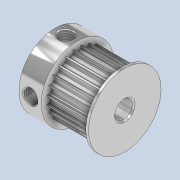
# Autodesk Inventor part: M6.35 24Tooth 15mm Deep 3M Timing Pulley
Saved by Autodesk Inventor 2022 (Build 260153000, 153)
## iProperties
Created: 2021-10-10
Part Number: M6.35 24Tooth 15mm Deep 3M Timing Pulley
Material: Generic
Document SubType Name: Modeling
Designer: Coy
Density: 1 g/cm^3
Appearance: Chrome - Polished
Author: Coy
Autodesk Inventor part; units mm, degrees
ref_plane "YZ Plane" through (0, 0, 0) normal (1, 0, 0) x (0, 1, 0)
sketch "Sketch1" plane through (0, 0, 0) normal (1, 0, 0) x (0, 1, 0)
  circle A0 centre (0, 0) radius 3.175
  circle A1 centre (0, 0) radius 13
  dimension "d0" = 6.35
  dimension "d1" = 26
  constraints: 2 centre point, 2 coincident
  measures "d0" diameter of A0
  measures "d1" diameter of A1
extrude "Extrusion1" add sketch "Sketch1" along normal blind 8
sketch "Sketch2" plane through (8, 0, 0) normal (1, 0, 0) x (0, 0, -1)
  circle A0 centre (0, 0) radius 3.175
  circle A1 centre (0, 0) radius 11.08
  line L0 (-1.45, 14.5114) -> (-1.45, 7.0707) construction
  line L1 (1.45, 14.5114) -> (1.45, 7.0707) construction
  arc A2 (-1.2, 10.18) -> (1.2, 10.18) centre (0, 11.08) ccw
  line L2 (1.2, 11.0148) -> (1.2, 10.18)
  line L3 (-1.2, 11.0148) -> (-1.2, 10.18)
  line L4 (-4.01, 10.3289) -> (-3.7939, 9.5225)
  arc A3 (-3.7939, 9.5225) -> (-1.4757, 10.1437) centre (-2.8677, 10.7025) ccw
  line L5 (-1.6917, 10.9501) -> (-1.4757, 10.1437)
  line L6 (-6.5466, 8.9391) -> (-6.1292, 8.2161)
  arc A4 (-6.1292, 8.2161) -> (-4.0508, 9.4161) centre (-5.54, 9.5956) ccw
  line L7 (-4.4682, 10.1391) -> (-4.0508, 9.4161)
  line L8 (-8.6372, 6.9401) -> (-8.0469, 6.3498)
  arc A5 (-8.0469, 6.3498) -> (-6.3498, 8.0469) centre (-7.8347, 7.8347) ccw
  line L9 (-6.9401, 8.6372) -> (-6.3498, 8.0469)
  line L10 (-10.1391, 4.4682) -> (-9.4161, 4.0508)
  arc A6 (-9.4161, 4.0508) -> (-8.2161, 6.1292) centre (-9.5956, 5.54) ccw
  line L11 (-8.9391, 6.5466) -> (-8.2161, 6.1292)
  line L12 (-10.9501, 1.6917) -> (-10.1437, 1.4757)
  arc A7 (-10.1437, 1.4757) -> (-9.5225, 3.7939) centre (-10.7025, 2.8677) ccw
  line L13 (-10.3289, 4.01) -> (-9.5225, 3.7939)
  line L14 (-11.0148, -1.2) -> (-10.18, -1.2)
  arc A8 (-10.18, -1.2) -> (-10.18, 1.2) centre (-11.08, 0) ccw
  line L15 (-11.0148, 1.2) -> (-10.18, 1.2)
  line L16 (-10.3289, -4.01) -> (-9.5225, -3.7939)
  arc A9 (-9.5225, -3.7939) -> (-10.1437, -1.4757) centre (-10.7025, -2.8677) ccw
  line L17 (-10.9501, -1.6917) -> (-10.1437, -1.4757)
  line L18 (-8.9391, -6.5466) -> (-8.2161, -6.1292)
  arc A10 (-8.2161, -6.1292) -> (-9.4161, -4.0508) centre (-9.5956, -5.54) ccw
  line L19 (-10.1391, -4.4682) -> (-9.4161, -4.0508)
  line L20 (-6.9401, -8.6372) -> (-6.3498, -8.0469)
  arc A11 (-6.3498, -8.0469) -> (-8.0469, -6.3498) centre (-7.8347, -7.8347) ccw
  line L21 (-8.6372, -6.9401) -> (-8.0469, -6.3498)
  line L22 (-4.4682, -10.1391) -> (-4.0508, -9.4161)
  arc A12 (-4.0508, -9.4161) -> (-6.1292, -8.2161) centre (-5.54, -9.5956) ccw
  line L23 (-6.5466, -8.9391) -> (-6.1292, -8.2161)
  line L24 (-1.6917, -10.9501) -> (-1.4757, -10.1437)
  arc A13 (-1.4757, -10.1437) -> (-3.7939, -9.5225) centre (-2.8677, -10.7025) ccw
  line L25 (-4.01, -10.3289) -> (-3.7939, -9.5225)
  line L26 (1.2, -11.0148) -> (1.2, -10.18)
  arc A14 (1.2, -10.18) -> (-1.2, -10.18) centre (0, -11.08) ccw
  line L27 (-1.2, -11.0148) -> (-1.2, -10.18)
  line L28 (4.01, -10.3289) -> (3.7939, -9.5225)
  arc A15 (3.7939, -9.5225) -> (1.4757, -10.1437) centre (2.8677, -10.7025) ccw
  line L29 (1.6917, -10.9501) -> (1.4757, -10.1437)
  line L30 (6.5466, -8.9391) -> (6.1292, -8.2161)
  arc A16 (6.1292, -8.2161) -> (4.0508, -9.4161) centre (5.54, -9.5956) ccw
  line L31 (4.4682, -10.1391) -> (4.0508, -9.4161)
  line L32 (8.6372, -6.9401) -> (8.0469, -6.3498)
  arc A17 (8.0469, -6.3498) -> (6.3498, -8.0469) centre (7.8347, -7.8347) ccw
  line L33 (6.9401, -8.6372) -> (6.3498, -8.0469)
  line L34 (10.1391, -4.4682) -> (9.4161, -4.0508)
  arc A18 (9.4161, -4.0508) -> (8.2161, -6.1292) centre (9.5956, -5.54) ccw
  line L35 (8.9391, -6.5466) -> (8.2161, -6.1292)
  line L36 (10.9501, -1.6917) -> (10.1437, -1.4757)
  arc A19 (10.1437, -1.4757) -> (9.5225, -3.7939) centre (10.7025, -2.8677) ccw
  line L37 (10.3289, -4.01) -> (9.5225, -3.7939)
  line L38 (11.0148, 1.2) -> (10.18, 1.2)
  arc A20 (10.18, 1.2) -> (10.18, -1.2) centre (11.08, 0) ccw
  line L39 (11.0148, -1.2) -> (10.18, -1.2)
  line L40 (10.3289, 4.01) -> (9.5225, 3.7939)
  arc A21 (9.5225, 3.7939) -> (10.1437, 1.4757) centre (10.7025, 2.8677) ccw
  line L41 (10.9501, 1.6917) -> (10.1437, 1.4757)
  line L42 (8.9391, 6.5466) -> (8.2161, 6.1292)
  arc A22 (8.2161, 6.1292) -> (9.4161, 4.0508) centre (9.5956, 5.54) ccw
  line L43 (10.1391, 4.4682) -> (9.4161, 4.0508)
  line L44 (6.9401, 8.6372) -> (6.3498, 8.0469)
  arc A23 (6.3498, 8.0469) -> (8.0469, 6.3498) centre (7.8347, 7.8347) ccw
  line L45 (8.6372, 6.9401) -> (8.0469, 6.3498)
  line L46 (4.4682, 10.1391) -> (4.0508, 9.4161)
  arc A24 (4.0508, 9.4161) -> (6.1292, 8.2161) centre (5.54, 9.5956) ccw
  line L47 (6.5466, 8.9391) -> (6.1292, 8.2161)
  line L48 (1.6917, 10.9501) -> (1.4757, 10.1437)
  arc A25 (1.4757, 10.1437) -> (3.7939, 9.5225) centre (2.8677, 10.7025) ccw
  line L49 (4.01, 10.3289) -> (3.7939, 9.5225)
  dimension "d4" = 22.16
  dimension "d5" = 1.45
  dimension "d6" = 1.45
  dimension "d7" = 3
  dimension "d8" = 0.25
  dimension "d9" = 0.25
  dimension "d10" = 11.08
  dimension "d13" = 360
  constraints: 100 end point, 48 point on circle, 25 centre point, 2 coincident, 2 parallel, 2 vertical, 197 other
  measures "d5" distance from line of point (0, 0) L1
  measures "d6" distance from line of point (0, 0) L0
  measures "d7" diameter of A2
  measures "d8" distance between parallel lines of L1 L2
  measures "d9" distance between parallel lines of L0 L3
  measures "d10" distance of point (0, 0) A2.centre
extrude "Extrusion2" add sketch "Sketch2" along normal blind 16 contours L38 A20 L39 A1 L36 A19 L37 L34 A18 L35 L32 A17 L33 L30 A16 L31 L28 A15 L29 L26 A14 L27 L24 A13 L25 L22 A12 L23 L20 A11 L21 L18 A10 L19 L16 A9 L17 L14 A8 L15 L12 A7 L13 L10 A6 L11 L8 A5 L9 L6 A4 L7 L4 A3 L5 L3 A2 L2 L48 A25 L49 L46 A24 L47 L44 A23 L45 L42 A22 L43 L40 A21 L41
sketch "Sketch3" plane through (24, 0, 0) normal (1, 0, 0) x (0, 0, -1)
  circle A0 centre (0, 0) radius 13 projected
  circle A1 centre (0, 0) radius 3.175 projected
extrude "Extrusion3" add sketch "Sketch3" along normal blind 1
chamfer "Chamfer1" distance 0.5 angle 45 2 edges at (25, 0, 3.175) (0, -3.175, 0)
ref_plane "Work Plane1" through (0, 13, 0) normal (0, 1, 0) x (-1, 0, 0)
sketch "Sketch4" plane through (0, 13, 0) normal (0, 1, 0) x (-1, 0, 0)
  line L0 (0, 0) -> (-8, 0) construction
  line L1 (-8, 13) -> (-8, -13) construction
  circle A0 centre (-4, 0) radius 2.5
  dimension "d23" = 5
  constraints: 2 end point, 2 midpoint, 1 centre point
  measures "d23" diameter of A0
extrude "Extrusion4" cut sketch "Sketch4" against normal up to next
ref_plane "Work Plane2" through (0, 0, 13) normal (0, 0, 1) x (1, 0, 0)
sketch "Sketch5" plane through (0, 0, 13) normal (0, 0, 1) x (1, 0, 0)
  line L0 (0, 0) -> (8, 0) construction
  line L1 (8, -13) -> (8, 13) construction
  circle A0 centre (4, 0) radius 2.5
  dimension "d27" = 5
  constraints: 2 end point, 2 midpoint, 1 centre point
  measures "d27" diameter of A0
extrude "Extrusion5" cut sketch "Sketch5" against normal up to next
chamfer "Chamfer2" distance 0.3 angle 45 4 edges at (4, 12.7574, 2.5) (4.0004, 12.7574, -2.5) (4.0039, 2.5, 12.7574) (3.7459, -2.4871, 12.7599)
thread "Thread1" size "M5x0.8" class "6H" standard "ANSI Metric M Profile" full length
thread "Thread2" size "M5x0.8" class "6H" standard "ANSI Metric M Profile" full length
equation "\"d6\" = d5"
equation "\"d10\" = 0.5 * d4"
body "Solid1"
